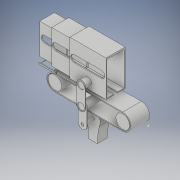
# Autodesk Inventor part: Collecter Arm Version 1
Saved by Autodesk Inventor 2019 (Build 230136000, 136)
## iProperties
Created: 2019-01-14
Part Number: Collecter Arm Version 1
Material: Generic
Document SubType Name: Modeling
Designer: mrhftc
Density: 1 g/cm^3
Appearance: Default
Author: mrhftc
Autodesk Inventor part; units mm, degrees
ref_plane "YZ Plane" through (0, 0, 0) normal (1, 0, 0) x (0, 1, 0)
ref_plane "XZ Plane" through (0, 0, 0) normal (0, 1, 0) x (-1, 0, 0)
ref_plane "XY Plane" through (0, 0, 0) normal (0, 0, 1) x (1, 0, 0)
sketch "Sketch1" plane through (0, 0, 0) normal (0, 1, 0) x (-1, 0, 0)
  line L0 (0, 0) -> (32.4478, 0)
  line L1 (32.4478, 0) -> (32.4478, 7.1949)
  line L2 (32.4478, 7.1949) -> (0, 7.1949)
  line L3 (0, 7.1949) -> (0, 0)
  constraints: 8 end point, 2 parallel, 1 horizontal, 1 perpendicular
extrude "Extrusion1" add sketch "Sketch1" along normal blind 6.35
fillet "Fillet1" radius 3.175 4 edges at (0, 6.35, 3.5975) (0, 0, 3.5975) (-32.4478, 6.35, 3.5975) (-32.4478, 0, 3.5975)
sketch "Sketch2" plane through (-29.2728, 0, 7.1949) normal (0, 0, 1) x (1, 0, 0)
  arc A0 (0, 6.35) -> (0, 0) centre (0, 3.175) ccw construction
  arc A1 (26.0978, 0) -> (26.0978, 6.35) centre (26.0978, 3.175) ccw construction
  arc A2 (0.0294, 6.0267) -> (-0.002, 0.3232) centre (0, 3.175) ccw
  arc A3 (26.0939, 0.3052) -> (26.0958, 6.0448) centre (26.0978, 3.175) ccw
  line L0 (-0.0334, 6.0266) -> (26.0958, 6.0448)
  line L1 (26.0978, 0.3052) -> (-0.002, 0.3232)
  point P0 (29.2728, 0)
  constraints: 6 point on circle, 4 end point, 2 centre point, 2 coincident, 2 point on line, 2 tangent
extrude "Extrusion2" cut sketch "Sketch2" against normal blind 6.731
sketch "Sketch3" plane through (-29.2728, 0, 0.4639) normal (0, 0, 1) x (1, 0, 0)
  arc A0 (-0.0334, 6.0266) -> (-0.002, 0.3232) centre (0, 3.175) ccw construction
  arc A1 (26.0978, 0.3052) -> (26.0958, 6.0448) centre (26.0978, 3.175) ccw construction
  circle A2 centre (0, 3.175) radius 2.616
  circle A3 centre (26.0978, 3.175) radius 2.616
  point P0 (29.2728, 0)
  constraints: 2 centre point, 2 coincident
extrude "Extrusion3" add sketch "Sketch3" along normal blind 6.731
sketch "Sketch4" plane through (-29.2728, 0, 0.4639) normal (0, 0, 1) x (1, 0, 0)
  circle A0 centre (13.0312, 3.176) radius 1.3351
  point P0 (29.2728, 0)
  constraints: 1 centre point
extrude "Extrusion4" add sketch "Sketch4" along normal blind 8.89
sketch "Sketch5" plane through (-16.2416, 3.176, 9.3539) normal (0, 0, 1) x (1, 0, 0)
  circle A0 centre (0, 0) radius 1.3351 construction
  arc A1 (1.6333, 0) -> (-1.6333, 0) centre (0, 0) ccw
  line L0 (1.6333, 0) -> (1.6333, -6.274)
  line L1 (-1.6333, -6.274) -> (-1.6333, 0)
  arc A2 (-1.6333, -6.274) -> (1.6333, -6.274) centre (0, -6.274) ccw
  circle A3 centre (0, 0) radius 1.3351 construction
  circle A4 centre (0, 0) radius 1.3351
  point P0 (16.2416, -3.176)
  constraints: 4 end point, 4 point on circle, 3 centre point, 2 coincident, 1 parallel
extrude "Extrusion5" add sketch "Sketch5" along normal blind 0.254
sketch "Sketch6" plane through (-16.2416, 3.176, 9.3539) normal (0, 0, -1) x (-1, 0, 0)
  arc A0 (-1.6333, -6.274) -> (1.6333, -6.274) centre (0, -6.274) ccw construction
  circle A1 centre (0, -6.274) radius 0.5616
  point P0 (-16.2416, -3.176)
  constraints: 1 centre point, 1 coincident
extrude "Extrusion6" add sketch "Sketch6" along normal blind 3.81
sketch "Sketch7" plane through (-16.2416, -3.098, 5.5439) normal (0, 0, -1) x (-1, 0, 0)
  circle A0 centre (0, 0) radius 0.5616 construction
  arc A1 (2.4069, -1.3892) -> (-2.4069, -1.3892) centre (0, 0) ccw
  arc A2 (-1.6333, 0) -> (1.6333, 0) centre (0, 0) ccw construction
  line L0 (1.6333, -7.627) -> (-1.6333, -7.627)
  arc A3 (2.4069, -1.3892) -> (1.6333, -7.627) centre (29.5953, -7.9278) ccw
  circle A4 centre (0, 0) radius 0.5616 construction
  line L1 (0, 0) -> (0, -1.6333) construction
  arc A5 (-1.6333, -7.627) -> (-2.4069, -1.3892) centre (-29.5953, -7.9278) ccw
  line L2 (-1.6333, 0) -> (-0.5616, 0)
  line L3 (0, 0) -> (0.5616, 0)
  point P0 (-16.2416, 3.098)
  point P1 (2.779, 0)
  point P2 (-2.779, 0)
  constraints: 10 point on circle, 8 end point, 3 centre point, 2 horizontal, 2 parallel, 2 symmetric about line, 1 coincident, 1 vertical, 1 other
extrude "Extrusion7" add sketch "Sketch7" along normal blind 3.81
sketch "Sketch8" plane through (-16.2416, 3.176, 9.3539) normal (0, 0, 1) x (1, 0, 0)
  circle A0 centre (0, 0) radius 1.3351 construction
  circle A1 centre (0, 0) radius 1.3351
  point P0 (16.2416, -3.176)
  constraints: 1 centre point, 1 coincident, 1 concentric
extrude "Extrusion8" add sketch "Sketch8" along normal blind 0.635
sketch "Sketch9" plane through (-16.2416, 3.176, 9.9889) normal (0, 0, 1) x (1, 0, 0)
  circle A0 centre (0, 0) radius 1.3351 construction
  line L0 (1.6333, -6.274) -> (1.6333, 0) construction
  arc A1 (-1.6333, 0) -> (1.6333, 0) centre (0, 0) ccw
  line L1 (1.6333, 0) -> (1.6333, 7.0513)
  line L2 (-1.6333, 7.0513) -> (-1.6333, 0)
  arc A2 (1.6333, 7.0513) -> (-1.6333, 7.0513) centre (0, 7.0513) ccw
  circle A3 centre (0, 7.0513) radius 1.3351
  circle A4 centre (0, 0) radius 1.3351
  point P0 (16.2416, -3.176)
  constraints: 5 point on circle, 4 centre point, 4 end point, 3 coincident, 1 parallel
extrude "Extrusion9" add sketch "Sketch9" along normal blind 0.254
sketch "Sketch10" plane through (-16.2416, 3.176, 9.9889) normal (0, 0, -1) x (-1, 0, 0)
  circle A0 centre (0, 7.0513) radius 1.3351 construction
  arc A1 (1.6333, 7.0513) -> (-1.6333, 7.0513) centre (0, 7.0513) ccw construction
  circle A2 centre (0, 7.0513) radius 1.3351
  point P0 (-16.2416, -3.176)
  constraints: 1 centre point, 1 coincident, 1 concentric
extrude "Extrusion10" add sketch "Sketch10" along normal blind 2.54
sketch "Sketch11" plane through (-16.2416, 3.176, 9.6079) normal (0, 0, 1) x (1, 0, 0)
  circle A0 centre (0, -6.274) radius 0.5616 construction
  circle A1 centre (0, -6.274) radius 0.5616
  point P0 (16.2416, -3.176)
  constraints: 1 centre point, 1 coincident
extrude "Extrusion11" cut sketch "Sketch11" against normal blind 0.254
sketch "Sketch12" plane through (-16.2416, 10.2273, 7.4489) normal (0, 0, -1) x (-1, 0, 0)
  line L0 (-6.8841, 10.5484) -> (7.0114, 10.5484)
  line L1 (7.0114, 10.5484) -> (7.0114, -2.6405)
  line L2 (7.0114, -2.6405) -> (-6.8841, -2.6405)
  line L3 (-6.8841, -2.6405) -> (-6.8841, 10.5484)
  point P0 (-16.2416, -10.2273)
  constraints: 8 end point, 2 parallel, 1 horizontal, 1 perpendicular
extrude "Extrusion12" add sketch "Sketch12" along normal blind 7.366
sketch "Sketch13" plane through (-23.253, 7.5868, 7.4489) normal (-1, 0, 0) x (0, 0, 1)
  line L0 (0, 13.1889) -> (-7.366, 13.1889) construction
  line L1 (-6.9628, 13.1889) -> (-0.3684, 13.1889)
  line L2 (-0.3684, 13.1889) -> (-0.3684, 0.2889)
  line L3 (-0.3684, 0.2889) -> (-6.9628, 0.2889)
  line L4 (-6.9628, 0.2889) -> (-6.9628, 13.1889)
  point P0 (-7.4489, -7.5868)
  constraints: 8 end point, 2 parallel, 1 horizontal, 1 perpendicular, 1 point on line
extrude "Extrusion13" cut sketch "Sketch13" against normal through all
sketch "Sketch14" plane through (-23.253, 7.5868, 7.4489) normal (-1, 0, 0) x (0, 0, 1)
  line L0 (-6.9628, 13.1889) -> (-0.3684, 13.1889)
  line L1 (-0.3684, 13.1889) -> (-0.3684, 0.2889)
  line L2 (-0.3684, 0.2889) -> (-6.9628, 0.2889)
  line L3 (-6.9628, 0.2889) -> (-6.9628, 13.1889)
  point P0 (-7.4489, -7.5868)
  constraints: 8 end point, 2 parallel, 1 horizontal, 1 perpendicular
extrude "Extrusion14" add sketch "Sketch14" along normal blind 7.366
sketch "Sketch15" plane through (-30.619, 7.5868, 7.4489) normal (-1, 0, 0) x (0, 0, 1)
  line L0 (-0.3684, 13.1889) -> (-6.9628, 13.1889) construction
  line L1 (-6.4971, 13.1889) -> (-0.8172, 13.1889)
  line L2 (-0.8172, 13.1889) -> (-0.8172, 0.7832)
  line L3 (-0.8172, 0.7832) -> (-6.4971, 0.7832)
  line L4 (-6.4971, 0.7832) -> (-6.4971, 13.1889)
  point P0 (-7.4489, -7.5868)
  constraints: 8 end point, 2 parallel, 1 horizontal, 1 perpendicular, 1 point on line
extrude "Extrusion15" cut sketch "Sketch15" against normal blind 7.366
sketch "Sketch16" plane through (-30.619, 7.5868, 7.4489) normal (-1, 0, 0) x (0, 0, 1)
  line L0 (-6.4971, 13.1889) -> (-0.8172, 13.1889)
  line L1 (-0.8172, 13.1889) -> (-0.8172, 0.7832)
  line L2 (-0.8172, 0.7832) -> (-6.4971, 0.7832)
  line L3 (-6.4971, 0.7832) -> (-6.4971, 13.1889)
  point P0 (-7.4489, -7.5868)
  constraints: 8 end point, 2 parallel, 1 horizontal, 1 perpendicular
extrude "Extrusion16" add sketch "Sketch16" along normal blind 5.08
sketch "Sketch17" plane through (-35.699, 7.5868, 7.4489) normal (-1, 0, 0) x (0, 0, 1)
  line L0 (-0.8172, 13.1889) -> (-6.4971, 13.1889) construction
  line L1 (-6.0679, 13.1889) -> (-1.184, 13.1889)
  line L2 (-1.184, 13.1889) -> (-1.184, 1.1108)
  line L3 (-1.184, 1.1108) -> (-6.0679, 1.1108)
  line L4 (-6.0679, 1.1108) -> (-6.0679, 13.1889)
  point P0 (-7.4489, -7.5868)
  constraints: 8 end point, 2 parallel, 1 horizontal, 1 perpendicular, 1 point on line
extrude "Extrusion17" cut sketch "Sketch17" against normal blind 5.08
sketch "Sketch18" plane through (-16.2416, 10.2273, 7.4489) normal (0, 0, 1) x (1, 0, 0)
  line L0 (5.1131, 6.2542) -> (-5.3164, 6.2542)
  line L1 (-5.3164, 3.5589) -> (5.1131, 3.5589)
  line L2 (-7.0114, -1.8573) -> (-7.0114, 10.5484) construction
  line L3 (-12.1131, 6.2542) -> (-7.0114, 6.2542)
  line L4 (-7.0114, 6.2542) -> (-7.0114, 3.5589)
  line L5 (-7.0114, 3.5589) -> (-12.1131, 3.5589)
  line L6 (-14.3774, -1.8573) -> (-14.3774, 10.5484) construction
  line L7 (-17.2693, 6.2542) -> (-14.3774, 6.2542)
  line L8 (-14.3774, 6.2542) -> (-14.3774, 3.5589)
  line L9 (-14.3774, 3.5589) -> (-17.2693, 3.5589)
  arc A0 (-17.2693, 6.2542) -> (-17.2693, 3.5589) centre (-17.2693, 4.9066) ccw
  arc A1 (-12.1131, 6.2542) -> (-12.1131, 3.5589) centre (-12.1131, 4.9066) ccw
  arc A2 (-5.3164, 6.2542) -> (-5.3164, 3.5589) centre (-5.3164, 4.9066) ccw
  arc A3 (5.1131, 3.5589) -> (5.1131, 6.2542) centre (5.1131, 4.9066) ccw
  point P0 (16.2416, -10.2273)
  constraints: 16 end point, 8 point on circle, 6 point on line, 4 centre point, 3 horizontal, 3 parallel, 2 perpendicular
extrude "Extrusion18" cut sketch "Sketch18" against normal blind 5.08 contours A3 L1 A2 L0
sketch "Sketch19" plane through (-23.253, 7.8757, 7.0806) normal (0, 0, 1) x (1, 0, 0)
  line L0 (0, 12.9) -> (0, 0) construction
  line L1 (0, 8.6058) -> (-5.7335, 8.6058)
  line L2 (-5.7335, 5.9121) -> (0, 5.9121)
  line L3 (0, 5.9121) -> (0, 8.6058)
  arc A0 (-5.7335, 8.6058) -> (-5.7335, 5.9121) centre (-5.7335, 7.259) ccw
  point P0 (23.253, -7.8757)
  constraints: 6 end point, 2 point on circle, 1 centre point, 1 horizontal, 1 parallel, 1 point on line
extrude "Extrusion19" cut sketch "Sketch19" against normal blind 5.08
sketch "Sketch20" plane through (-30.619, 8.3701, 6.6317) normal (0, 0, 1) x (1, 0, 0)
  line L0 (0, -0.4944) -> (0, 12.4057) construction
  line L1 (0, 5.4006) -> (-3.1642, 5.4006)
  line L2 (-3.1642, 7.9964) -> (0, 7.9964)
  line L3 (0, 7.9964) -> (0, 5.4006)
  arc A0 (-3.1642, 7.9964) -> (-3.1642, 5.4006) centre (-3.1642, 6.6985) ccw
  point P0 (30.619, -8.3701)
  constraints: 6 end point, 2 point on circle, 1 centre point, 1 horizontal, 1 parallel, 1 point on line
extrude "Extrusion20" cut sketch "Sketch20" against normal blind 5.08
sketch "Sketch21" plane through (-35.699, 20.7757, 0.9519) normal (0, 1, 0) x (1, 0, 0)
  line L0 (0, 0) -> (5.08, 0)
  line L1 (5.08, 0) -> (5.08, -0.4291)
  line L2 (5.08, -0.4291) -> (0, -0.4291)
  line L3 (0, -0.4291) -> (0, 0)
  line L4 (0, -5.3131) -> (0, -0.4291) construction
  line L5 (5.08, -5.6799) -> (5.08, -5.3131) construction
  line L6 (0, -5.3131) -> (5.08, -5.3131)
  line L7 (5.08, -5.3131) -> (5.08, -5.6799)
  line L8 (5.08, -5.6799) -> (0, -5.6799)
  line L9 (0, -5.6799) -> (0, -5.3131)
  line L10 (6.4242, 0.4879) -> (3.5743, 0.4879) construction
  line L11 (12.446, 0) -> (5.08, 0)
  line L12 (5.08, 0) -> (5.08, 0.4879)
  line L13 (5.08, 0.4879) -> (12.446, 0.4879)
  line L14 (12.446, 0.4879) -> (12.446, 0)
  line L15 (12.446, -5.6799) -> (12.446, -6.1287) construction
  line L16 (5.08, -6.1287) -> (5.08, -5.6799) construction
  line L17 (12.446, -5.6799) -> (5.08, -5.6799)
  line L18 (5.08, -5.6799) -> (5.08, -6.1287)
  line L19 (5.08, -6.1287) -> (12.446, -6.1287)
  line L20 (12.446, -6.1287) -> (12.446, -5.6799)
  point P0 (35.699, 0.9519)
  point P1 (6.3928, 0.4879)
  constraints: 32 end point, 8 parallel, 4 horizontal, 4 perpendicular, 2 point on line
extrude "Extrusion21" cut sketch "Sketch21" against normal blind 0.635
sketch "Sketch22" plane through (-35.699, 20.1407, 0.9519) normal (0, 1, 0) x (1, 0, 0)
  line L0 (0, 0) -> (5.08, 0)
  line L1 (5.08, 0) -> (5.08, -0.4291)
  line L2 (5.08, -0.4291) -> (0, -0.4291)
  line L3 (0, -0.4291) -> (0, 0)
  line L4 (0, -5.3131) -> (5.08, -5.3131) construction
  line L5 (5.08, -5.6799) -> (12.446, -5.6799) construction
  line L6 (0, -5.3131) -> (5.08, -5.3131)
  line L7 (5.08, -5.3131) -> (5.08, -5.6799)
  line L8 (5.08, -5.6799) -> (0, -5.6799)
  line L9 (0, -5.6799) -> (0, -5.3131)
  point P0 (35.699, 0.9519)
  constraints: 16 end point, 4 parallel, 2 horizontal, 2 perpendicular
extrude "Extrusion22" cut sketch "Sketch22" against normal blind 0.635
sketch "Sketch23" plane through (-23.253, 20.7757, 0.0829) normal (0, 1, 0) x (1, 0, 0)
  line L0 (13.8954, -7.366) -> (0, -7.366) construction
  line L1 (0, 0) -> (13.8954, 0)
  line L2 (13.8954, 0) -> (13.8954, -7.366)
  line L3 (13.8954, -7.366) -> (0, -7.366)
  line L4 (0, -7.366) -> (0, 0)
  point P0 (23.253, 0.0829)
  constraints: 8 end point, 2 parallel, 1 horizontal, 1 perpendicular
extrude "Extrusion23" add sketch "Sketch23" along normal blind 0.635
sketch "Sketch24" plane through (-35.699, 20.1407, 0.9519) normal (0, 1, 0) x (1, 0, 0)
  line L0 (12.446, 0.4657) -> (5.08, 0.4657) construction
  line L1 (5.08, 0.4657) -> (12.446, 0.4657)
  line L2 (12.446, 0.4657) -> (12.446, -6.1287)
  line L3 (12.446, -6.1287) -> (5.08, -6.1287)
  line L4 (5.08, -6.1287) -> (5.08, 0.4657)
  point P0 (35.699, 0.9519)
  constraints: 8 end point, 2 parallel, 1 horizontal, 1 perpendicular
extrude "Extrusion24" add sketch "Sketch24" along normal blind 0.635
sketch "Sketch25" plane through (-35.699, 19.5057, 0.9519) normal (0, 1, 0) x (1, 0, 0)
  line L0 (0, 0) -> (0, -5.6799) construction
  line L1 (0, 0) -> (5.08, 0)
  line L2 (5.08, 0) -> (5.08, -5.6799)
  line L3 (5.08, -5.6799) -> (0, -5.6799)
  line L4 (0, -5.6799) -> (0, 0)
  point P0 (35.699, 0.9519)
  constraints: 8 end point, 2 parallel, 1 horizontal, 1 perpendicular
extrude "Extrusion25" add sketch "Sketch25" along normal blind 0.635
sketch "Sketch26" plane through (-9.3575, 7.5868, 7.4489) normal (1, 0, 0) x (0, 0, -1)
  line L0 (0, 0) -> (7.366, 0) construction
  line L1 (6.0679, 1.1108) -> (1.184, 1.1108) construction
  line L2 (4.5126, 0) -> (2.8745, 0)
  line L3 (2.8745, 0) -> (2.8745, 1.1108)
  line L4 (2.8745, 1.1108) -> (4.5126, 1.1108)
  line L5 (4.5126, 1.1108) -> (4.5126, 0)
  point P0 (7.4489, -7.5868)
  constraints: 8 end point, 2 parallel, 2 point on line, 1 horizontal, 1 perpendicular
extrude "Extrusion26" cut sketch "Sketch26" against normal through all
sketch "Sketch27" plane through (-30.619, 8.3701, 4.5744) normal (0, 0, -1) x (-1, 0, 0)
  line L0 (0, 0.3276) -> (5.08, 0.3276) construction
  line L1 (3.3156, 0.3276) -> (4.7286, 0.3276)
  line L2 (4.7286, 0.3276) -> (4.7286, -0.7799)
  line L3 (3.3156, -0.7799) -> (3.3156, 0.3276)
  arc A0 (3.3156, -0.7799) -> (4.7286, -0.7799) centre (4.0221, -0.7799) ccw
  point P0 (-30.619, -8.3701)
  constraints: 6 end point, 2 point on circle, 1 centre point, 1 horizontal, 1 parallel, 1 perpendicular, 1 point on line
extrude "Extrusion27" add sketch "Sketch27" along normal blind 0.254
sketch "Sketch28" plane through (-30.619, 8.3701, 4.5744) normal (0, 0, 1) x (1, 0, 0)
  arc A0 (-4.7286, -0.7799) -> (-3.3156, -0.7799) centre (-4.0221, -0.7799) ccw construction
  arc A1 (-4.0983, -1.3843) -> (-3.9458, -1.3843) centre (-4.0221, -0.7799) ccw
  arc A2 (-3.9458, -1.3843) -> (-4.0983, -1.3843) centre (-4.0221, -1.2441) ccw
  point P0 (30.619, -8.3701)
  constraints: 4 point on circle, 2 centre point, 1 coincident
extrude "Extrusion28" add sketch "Sketch28" along normal blind 3.048
sketch "Sketch29" plane through (-30.619, 8.3701, 7.6224) normal (0, 0, 1) x (1, 0, 0)
  arc A0 (-3.9458, -1.3843) -> (-4.0983, -1.3843) centre (-4.0221, -1.2441) ccw construction
  line L0 (-4.0221, -0.9946) -> (1.816, -0.9946)
  line L1 (1.816, -1.4916) -> (-4.0221, -1.4916)
  arc A1 (-4.0221, -0.9946) -> (-3.991, -1.4916) centre (-4.0221, -1.2441) ccw
  arc A2 (1.816, -1.4916) -> (1.816, -0.9946) centre (1.816, -1.2431) ccw
  point P0 (30.619, -8.3701)
  constraints: 4 end point, 4 point on circle, 2 centre point, 1 coincident, 1 horizontal, 1 parallel, 1 point on line
extrude "Extrusion29" add sketch "Sketch29" along normal blind 0.254
sketch "Sketch30" plane through (-30.619, 8.3701, 7.6224) normal (0, 0, -1) x (-1, 0, 0)
  arc A0 (-1.816, -0.9946) -> (-1.816, -1.4916) centre (-1.816, -1.2431) ccw construction
  circle A1 centre (-1.816, -1.2431) radius 0.1845
  point P0 (-30.619, -8.3701)
  constraints: 1 centre point, 1 coincident
extrude "Extrusion30" add sketch "Sketch30" along normal blind 0.4064
sketch "Sketch31" plane through (-28.8029, 7.1269, 7.216) normal (0, 0, -1) x (-1, 0, 0)
  circle A0 centre (0, 0) radius 0.1845 construction
  line L0 (-25.6279, -0.7769) -> (0.4699, -0.7769) construction
  line L1 (0.1845, 0) -> (0.1845, -0.7769)
  line L2 (0.1845, -0.7769) -> (-0.1845, -0.7769)
  line L3 (-0.1845, -0.7769) -> (-0.1845, 0)
  arc A1 (0.1845, 0) -> (-0.1845, 0) centre (0, 0) ccw
  point P0 (-28.8029, -7.1269)
  constraints: 6 end point, 2 point on circle, 1 centre point, 1 coincident, 1 horizontal alignment, 1 parallel, 1 point on line, 1 other
extrude "Extrusion31" add sketch "Sketch31" along normal blind 0.0762
sketch "Sketch32" plane through (-29.2728, 0, 0.4639) normal (0, 0, 1) x (1, 0, 0)
  circle A0 centre (13.0312, 3.176) radius 1.3351 construction
  circle A1 centre (0, 3.175) radius 2.616 construction
  circle A2 centre (26.0978, 3.175) radius 2.616 construction
  arc A3 (-0.0334, 6.0266) -> (-0.002, 0.3232) centre (0, 3.175) ccw construction
  line L0 (26.0978, 0.3052) -> (-0.002, 0.3232) construction
  arc A4 (26.0978, 0.3052) -> (26.0958, 6.0448) centre (26.0978, 3.175) ccw construction
  line L1 (-0.0334, 6.0266) -> (26.0958, 6.0448) construction
  circle A5 centre (0, 3.175) radius 2.616
  circle A6 centre (13.0312, 3.176) radius 1.3351
  circle A7 centre (26.0978, 3.175) radius 2.616
  point P0 (29.2728, 0)
  constraints: 3 centre point, 3 coincident, 1 concentric
body "Solid1"
